Autodesk Fusion 360 part; units mm, degrees
(part 2 of 2)
sketch "Sketch100" plane through (0, 0, 0) normal (0, 1, 0) x (-1, 0, 0)
  line L0 (-9.75, 10.558) -> (-33.75, 10.558)
  line L1 (-33.75, 10.558) -> (-33.75, 23.558)
  line L2 (-33.75, 23.558) -> (-9.75, 23.558)
  line L3 (-9.75, 23.558) -> (-9.75, 10.558)
  circle A0 centre (-88, 15) radius 7
  line L4 (-81, 15) -> (-81, 16)
  line L5 (-81, 16) -> (-37, 16)
  line L6 (-37, 16) -> (-37, 3)
  line L7 (-37, 3) -> (-81, 3)
  line L8 (-81, 3) -> (-81, 15)
  circle A1 centre (-64.5, 18.1) radius 1.625
  line L9 (-58.3, 29.3) -> (-36.7, 29.3)
  line L10 (-36.7, 29.3) -> (-36.7, 16.7)
  line L11 (-36.7, 16.7) -> (-58.3, 16.7)
  line L12 (-58.3, 16.7) -> (-58.3, 29.3)
  circle A2 centre (-72.5, 18.1) radius 1.625
  circle A3 centre (-33.5, 3.06) radius 1.5
  circle A4 centre (-33.5, 26.86) radius 1.5
  circle A5 centre (-10, 3.06) radius 1.5
  circle A6 centre (-10, 26.86) radius 1.5
  line L13 (1, 31) -> (-102.6, 31)
  line L14 (-102.6, 31) -> (-102.6, -1)
  line L15 (-102.6, -1) -> (1, -1)
  line L16 (1, -1) -> (1, 31)
  line L17 (-3, 30) -> (-3, 3)
  line L18 (-14.9874, 3) -> (-3, 3)
  line L19 (-98.6, 30) -> (-98.6, 3)
  line L20 (-98.6, 3) -> (-79.9963, 3)
  line L21 (-3, 3) -> (-6, 3)
  line L22 (-6, 3) -> (-6, 29)
  line L23 (-6, 29) -> (-3, 29)
  line L24 (-3, 29) -> (-3, 3)
  line L25 (-98.6, 3) -> (-95.6, 3)
  line L26 (-95.6, 3) -> (-95.6, 29)
  line L27 (-95.6, 29) -> (-98.6, 29)
  line L28 (-98.6, 29) -> (-98.6, 3)
  dimension "d530" = 3
  constraint horizontal L21
  constraint vertical L22
  constraint horizontal L23
  constraint vertical L24
  constraint coincident L17.end L18.end
  constraint horizontal L25
  constraint vertical L26
  constraint horizontal L27
  constraint vertical L28
  constraint coincident L19.end L20.start
  measures "d530" distance of L19.end L25.end
extrude "Extrude67" add sketch "Sketch100" along normal blind 12 contours L17 L18 L21 L22 L23 L24 | L19 L20 L25 L26 L27 L28 bodies 4
box "BoxPrimitive16" add length 26 width 3 height 4 placed x (0, 0, 1) y (1, 0, 0) z (0, 1, 0) at (3, 12, 3) bodies 4
fillet "Fillet3" radius 5 2 edges at (4.5, 16, 3) (4.5, 16, 29) on bodies 4
fillet "Fillet4" radius 5 2 edges at (97.1, 12, 29) (97.1, 12, 3) on bodies 4
box "BoxPrimitive17" cut length 9 width 32 height -3 placed x (0, 1, 0) y (-1, 0, 0) z (0, 0, 1) at (38, 0, 3) bodies 7
chamfer "Chamfer17" distance 0.75 angle 45 1 edges at (32.6143, 5, 27.2035) on bodies 4
chamfer "Chamfer18" distance 0.75 angle 45 1 edges at (9.1143, 5, 27.2035) on bodies 4
chamfer "Chamfer19" distance 0.75 angle 45 1 edges at (32.6143, 5, 3.4035) on bodies 4
chamfer "Chamfer20" distance 0.75 angle 45 1 edges at (9.1143, 5, 3.4035) on bodies 4
hole "Hole26" at (98.6, 7, 24) direction (-1, 0, 0) diameter 3.5 depth 10 tip angle 118 bodies 4
hole "Hole27" at (98.6, 7, 8) direction (-1, 0, 0) diameter 3.5 depth 10 tip angle 118 bodies 4
hole "Hole28" at (3, 11, 24) direction (1, 0, 0) diameter 3.5 depth 10 tip angle 118 bodies 4
hole "Hole29" at (3, 11, 8) direction (1, 0, 0) diameter 3.5 depth 10 tip angle 118 bodies 4
hole "Hole31" at (6, 11, 8) direction (-1, 0, 0) diameter 3 depth 10 tip angle 118 bodies 7
hole "Hole32" at (6, 11, 24) direction (-1, 0, 0) diameter 3 depth 10 tip angle 118 bodies 7
hole "Hole33" at (95.6, 7, 24) direction (1, 0, 0) diameter 3 depth 10 tip angle 118 bodies 7
hole "Hole34" at (95.6, 7, 8) direction (1, 0, 0) diameter 3 depth 10 tip angle 118 bodies 7
sketch "Sketch103" plane through (98.6, 0, 0) normal (-1, 0, 0) x (0, -1, 0)
  line L0 (-115.4914, 3) -> (-115.4914, 4.7212)
  arc A0 (-106.5116, 5.3236) -> (-115.4914, 4.7212) centre (-111, 5) ccw
  line L1 (-106.5116, 5.3236) -> (-106.5116, 3)
  line L2 (-106.5116, 3) -> (-103.9762, 3)
  line L3 (-103.9762, 3) -> (-103.9762, 8)
  line L4 (-103.9762, 8) -> (-100.3095, 8)
  line L5 (-100.3095, 8) -> (-100.3095, 30)
  line L6 (-100.3095, 30) -> (-121, 30)
  line L7 (-121, 30) -> (-121, 3)
  line L8 (-121, 3) -> (-115.4914, 3)
  line L9 (-16, 30) -> (-35.799, 10.201)
  line L10 (-16, 30) -> (12, 30) construction
  line L11 (-34, 8) -> (-34, 11)
  line L12 (-34, 11) -> (-123, 12)
  line L13 (-16, 30) -> (-121, 30)
  line L14 (-121, 30) -> (-121, 12)
  dimension "d596" = 135
  dimension "d597" = 28
  constraint horizontal L10
  constraint vertical L11
  constraint coincident L6.end L7.start
  constraint coincident L7 L14.end
  constraint perpendicular L6 L14
  measures "d596" angle of L9 L10
  measures "d597" distance of L9.start L9.end
extrude "Extrude68" cut sketch "Sketch103" against normal blind 3 contours L5 L6 L7 L12 L13 L14 | L5 L9 L12 L13 bodies 7
sketch "Sketch104" plane through (0, 0, 0) normal (-1, 0, 0) x (0, -1, 0)
  circle A0 centre (-11, 24) radius 1.5
  circle A1 centre (-11, 8) radius 1.5
  circle A2 centre (-111, 5) radius 1.5
  circle A3 centre (-21, 5) radius 1.5
  line L0 (-121, 0) -> (0, 0)
  line L1 (0, 0) -> (0, 30)
  line L2 (0, 30) -> (-121, 30)
  line L3 (-121, 30) -> (-121, 0)
  line L4 (-16, 30) -> (-29.7311, 16.2689)
  line L5 (-34.9889, 11.0111) -> (-97.7718, 11.7165)
  line L6 (-16, 30) -> (-34.9889, 11.0111)
  line L7 (-16, 30) -> (-121, 30)
  line L8 (-97.7718, 11.7165) -> (-121, 11.7165)
  line L9 (-121, 30) -> (-121, 11.7165)
  constraint coincident L4.start L6.start
  constraint coincident L5.start L6.end
  constraint coincident L2.end L3.start
  constraint coincident L5.end L8.start
  constraint coincident L3 L8.end
  constraint perpendicular L3 L8
extrude "Extrude69" cut sketch "Sketch104" against normal blind 5 contours L2 L3 L4 L5 L6 L7 L8 L9 bodies 7
fillet "Fillet5" radius 5 6 edges at (100.1, 16, 30) (100.1, 34.9889, 11.0111) (100.1, 121, 11.9775) (1.5, 121, 11.7165) (1.5, 34.9889, 11.0111) (1.5, 16, 30) on bodies 7
fillet "Fillet6" radius 5 4 edges at (14.9874, 105, 1.5) (14.9874, 121, 1.5) (79.9963, 105, 1.5) (79.9963, 121, 1.5) on bodies 7
fillet "Fillet7" radius 5 2 edges at (38, 9, 1.5) (6, 9, 1.5) on bodies 7
fillet "Fillet8" radius 3 1 edges at (6, 0, 1.5) on bodies 7
fillet "Fillet9" radius 3 1 edges at (38, 0, 1.5) on bodies 7
equation "d326 = ( 12.864 / 2 ) * 1 mm"
named bodies: "Gotek Board", "Encoder", "OLED", "Front Panel", "USB Cover", "Knob", "Case"
